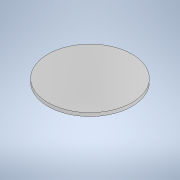
# Autodesk Inventor part: mirror001
Saved by Autodesk Inventor 2020 (Build 240168000, 168)
## iProperties
Created: 2024-01-27
Part Number: mirror001
Material: Алюминий 6061-AHC
Document SubType Name: Modeling
Designer: 4s
Density: 2.7 g/cm^3
Appearance: Алюминий — темный
Author: 4s
Autodesk Inventor part; units mm, degrees
ref_plane "YZ Plane" through (0, 0, 0) normal (1, 0, 0) x (0, 1, 0)
ref_plane "XZ Plane" through (0, 0, 0) normal (0, 1, 0) x (-1, 0, 0)
ref_plane "XY Plane" through (0, 0, 0) normal (0, 0, 1) x (1, 0, 0)
sketch "Эскиз1" plane through (0, 0, 0) normal (1, 0, 0) x (0, 1, 0)
  line L0 (0, 0) -> (82.3862, 0) construction
  line L1 (0, -22) -> (131.5712, -22)
  line L2 (0, 22) -> (131.5712, 22)
  line L3 (26.2186, 22) -> (26.2186, -22)
  line L4 (16.2186, 0) -> (26.2186, -22)
  line L5 (16.2186, 0) -> (26.2186, 22)
  line L6 (8.9501, -29.8493) -> (26.2186, -22)
  line L7 (26.2186, -22) -> (16.9413, -499.9139) construction
  line L8 (0, 0) -> (26.2186, -22) construction
  line L9 (0, 22) -> (0, -22) construction
  line L10 (0, 0) -> (26.2186, 22) construction
  line L11 (21.2186, -11) -> (3.6083, -19.0047) construction
  line L12 (0, 0) -> (21.2186, -11) construction
  line L13 (21.2186, -11) -> (-94.4642, -485.2171) construction
  line L14 (-6.7158, 12.3332) -> (16.9375, 1.5817) construction
  line L15 (0, 0) -> (16.9375, 1.5817) construction
  line L16 (-271.4302, 401.7527) -> (16.9375, 1.5817) construction
  circle A0 centre (26.2186, 0) radius 500 construction
  line L17 (-110, 105) -> (-60, 105) construction
  line L18 (-60, 105) -> (-60, -105) construction
  line L19 (-60, -105) -> (-110, -105) construction
  line L20 (-110, -105) -> (-110, 105) construction
  line L21 (-20, 47) -> (-60, 47) construction
  line L22 (-60, 47) -> (-60, -47) construction
  line L23 (-60, -47) -> (-20, -47) construction
  line L24 (-20, -47) -> (-20, 47) construction
  line L25 (16.2186, 0) -> (26.2186, 0)
  line L26 (26.2186, 22) -> (26.2186, 25)
  line L27 (26.2186, 25) -> (28.2186, 25)
  line L28 (26.2186, -22) -> (26.2186, -25)
  line L29 (26.2186, -25) -> (28.2186, -25)
  line L30 (28.2186, 25) -> (28.2186, -25)
  line L31 (26.2186, 0) -> (28.2186, 0)
  dimension "d1" = 178.888
  dimension "d2" = 80
  dimension "d3" = 26.2186
  dimension "d4" = 10
  dimension "d5" = 131.112
  dimension "d6" = 1000
  dimension "d7" = 44
  dimension "d8" = 50
  dimension "d9" = 210
  dimension "d10" = 40
  dimension "d11" = 94
  dimension "d13" = 20
  dimension "d14" = 136.2186
  dimension "d15" = 3
  dimension "d16" = 2
  dimension "d17" = 3
  dimension "d18" = 2
  constraints: 64 end point, 6 horizontal, 6 perpendicular, 5 point on line, 5 vertical, 4 midpoint, 4 parallel, 3 point on circle, 2 symmetric about line, 1 centre point, 1 collinear, 5 other
  measures "d1" angle of L3 L7
  measures "d2" angle of L10 L8
  measures "d3" distance from line of L3 L0.start
  measures "d4" distance from line of L3 L4.start
  measures "d5" angle of L5 L4
  measures "d6" diameter of A0
  measures "d7" distance of L3.start L3.end
  measures "d8" distance of L18.end L19.end
  measures "d9" distance of L17.end L18.end
  measures "d10" distance of L23.end L22.end
  measures "d11" distance of L22.end L21.end
  measures "d13" distance from line of L24 L0.start
  measures "d14" distance between parallel lines of L3 L20
  measures "d15" distance of L3.start L26.end
  measures "d16" distance of L26.end L27.end
  measures "d17" distance of L3.end L28.end
  measures "d18" distance of L28.end L29.end
revolve "Вращение1" add sketch "Эскиз1" angle 360 about axis through (0, 0, 0) along (0, 1, 0) contours L3 L31 L30 L1 | L4 L25 L3 | L1 L30 L29 L28
